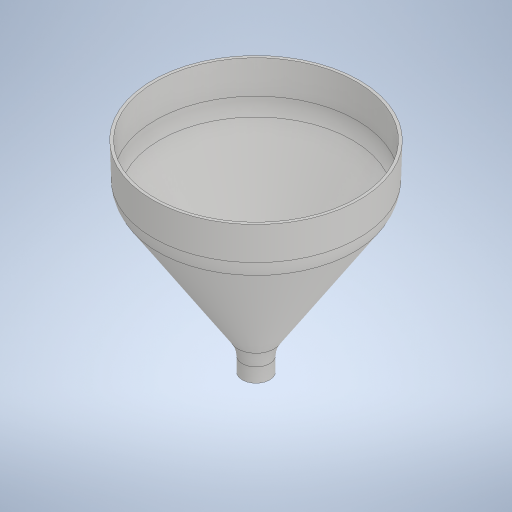
# Autodesk Inventor part: Funnel 2
Saved by Autodesk Inventor 2023 (Build 270158000, 158)
## iProperties
Created: 2020-02-13
Part Number: Funnel 2
Material: PET Plastic
Document SubType Name: Modeling
Designer: zachwan
Mass: 121.787 g
Surface Area: 1226.11 cm^2
Volume: 121.787 cm^3
Density: 1.541 g/cm^3
Appearance: Default
Author: zachwan
Autodesk Inventor part; units mm, degrees
ref_plane "YZ Plane" through (0, 0, 0) normal (1, 0, 0) x (0, 1, 0)
ref_plane "XZ Plane" through (0, 0, 0) normal (0, 1, 0) x (-1, 0, 0)
ref_plane "XY Plane" through (0, 0, 0) normal (0, 0, 1) x (1, 0, 0)
sketch "Sketch1" plane through (0, 0, 0) normal (0, 0, 1) x (1, 0, 0)
  line L0 (0, 0) -> (0, 20)
  line L1 (0, 0) -> (0, 145)
  line L2 (74.9981, 145.5303) -> (74.1596, 115.542)
  line L3 (10, 0) -> (10, 10.1792)
  line L4 (13.1928, 21.0198) -> (71.1308, 110.8462)
  line L5 (73, 145.5303) -> (73, 121.4795)
  line L6 (69.8072, 110.6389) -> (12.1928, 21.3144)
  line L7 (9, 10.4737) -> (9, 0)
  line L8 (9, 0) -> (10, 0)
  line L9 (73, 145.5303) -> (74.9981, 145.5303)
  arc A0 (69.8072, 110.6389) -> (73, 121.4795) centre (53, 121.4795) ccw
  arc A1 (71.1308, 110.8462) -> (74.3158, 121.1278) centre (54.3236, 121.6868) ccw
  arc A2 (13.1928, 21.0198) -> (10, 10.1792) centre (30, 10.1792) ccw
  arc A3 (12.1928, 21.3144) -> (9, 10.4737) centre (29, 10.4737) ccw
  dimension "d0" = 20
  dimension "d4" = 10
  dimension "d16" = 75
  dimension "d20" = 1
  dimension "d21" = 20
  dimension "d26" = 30
  dimension "d27" = 89.8263
  dimension "d28" = 106.8905
  dimension "d29" = 10.4738
  constraints: 20 end point, 8 point on circle, 5 tangent, 4 centre point, 3 equal radius, 3 vertical, 2 horizontal, 2 point on line, 1 other
  measures "d0" distance of L0.start L0.end
  measures "d4" distance of L0.start L3.start
  measures "d16" distance of L1.end L2.start
  measures "d20" distance between parallel lines of L4 L6
  measures "d21" radius of A0
  measures "d26" distance of L2.start L2.end
  measures "d27" vertical distance of L4.start L4.end
  measures "d28" distance of L4.start L4.end
  measures "d29" distance of L7.start L7.end
revolve "Revolution1" add sketch "Sketch1" angle 360 about axis through (0, 0, 0) along (0, 1, 0)
body "Solid1"
